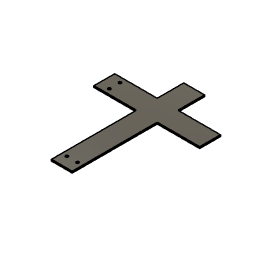
suporte (Autodesk Fusion 360 design; units mm, degrees)
Autodesk Fusion 360 part; units mm, degrees
sketch "Sketch1" plane through (0, 0, 0) normal (0, 0, 1) x (1, 0, 0)
  line L0 (0, 0) -> (40, 0)
  line L1 (40, 0) -> (40, 200)
  line L2 (40, 200) -> (0, 200)
  line L3 (0, 200) -> (0, 0)
  line L4 (40, 200) -> (120, 200)
  line L5 (120, 200) -> (120, 160)
  line L6 (120, 160) -> (40, 160)
  line L7 (40, 160) -> (40, 200)
  line L8 (0, 200) -> (-80, 200)
  line L9 (-80, 200) -> (-80, 160)
  line L10 (-80, 160) -> (0, 160)
  line L11 (0, 160) -> (0, 200)
  line L12 (0, 200) -> (40, 200)
  line L13 (40, 200) -> (40, 250)
  line L14 (40, 250) -> (0, 250)
  line L15 (0, 250) -> (0, 200)
  circle A0 centre (10, 20) radius 2
  circle A1 centre (30, 20) radius 2
  circle A2 centre (-60, 190) radius 2
  circle A3 centre (-60, 170) radius 2
  dimension "d1" = 40
  dimension "d2" = 200
  dimension "d3" = 80
  dimension "d4" = 40
  dimension "d5" = 80
  dimension "d6" = 40
  dimension "d7" = 4
  dimension "d8" = 4
  dimension "d9" = 4
  dimension "d10" = 4
  constraint horizontal L0
  constraint vertical L1
  constraint horizontal L2
  constraint vertical L3
  constraint coincident L0.start L3.end
  constraint horizontal L4
  constraint vertical L5
  constraint horizontal L6
  constraint vertical L7
  constraint horizontal L8
  constraint vertical L9
  constraint horizontal L10
  constraint vertical L11
  constraint horizontal L12
  constraint vertical L13
  constraint horizontal L14
  constraint vertical L15
  measures "d1" distance of L0.start L0.end
  measures "d2" distance of L0.start L2.end
  measures "d3" distance of L1.end L4.end
  measures "d4" distance of L1.end L6.end
  measures "d5" distance of L2.end L8.end
  measures "d6" distance of L2.end L10.end
  measures "d7" diameter of A0
  measures "d8" diameter of A1
  measures "d9" diameter of A2
  measures "d10" diameter of A3
extrude "Extrude1" add sketch "Sketch1" along normal blind 3
fillet "Fillet1" radius 0.5 18 faces at (26.6667, 250, 1) (93.3333, 160, 1) (23.3333, 114, 0) (40, 53.3333, 1) (13.3333, 0, 1) (0, 106.6667, 1) (-53.3333, 160, 1) (40, 216.6667, 1) (-58.0025, 170.0997, 1) (31.9975, 19.9003, 2) (-61.9603, 190.3963, 2) (66.6667, 200, 1) (11.9975, 19.9003, 2) (120, 186.6667, 1) (23.3333, 114, 3) (-80, 186.6667, 1) (0, 233.3333, 1) (-26.6667, 200, 1)
